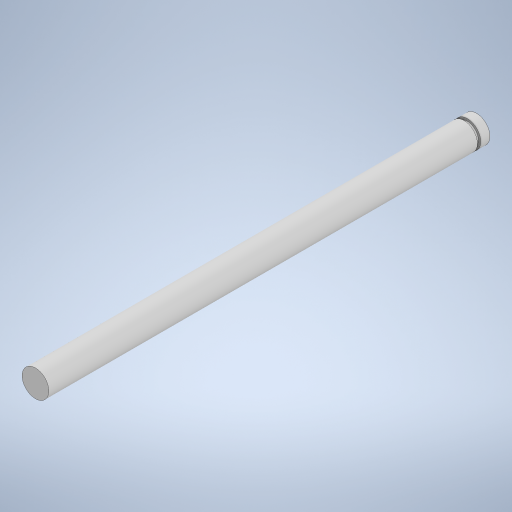
# Autodesk Inventor part: Eixo do Motor Industrial
Saved by Autodesk Inventor 2023 (Build 270158030, 158C)
## iProperties
Created: 2022-07-19
Part Number: Eixo do Motor Industrial
Material: Generic
Document SubType Name: Modeling
Designer: coqui
Density: 1 g/cm^3
Appearance: Default
Author: coqui
Autodesk Inventor part; units mm, degrees
ref_plane "YZ Plane" through (0, 0, 0) normal (1, 0, 0) x (0, 1, 0)
ref_plane "XZ Plane" through (0, 0, 0) normal (0, 1, 0) x (-1, 0, 0)
ref_plane "XY Plane" through (0, 0, 0) normal (0, 0, 1) x (1, 0, 0)
sketch "Sketch1" plane through (0, 0, 0) normal (0, 0, 1) x (1, 0, 0)
  circle A0 centre (0, 0) radius 7.25
  dimension "d0" = 14.5
  constraints: 1 centre point, 1 coincident
  measures "d0" diameter of A0
extrude "Extrusion1" add sketch "Sketch1" along normal blind 240
sketch "Sketch2" plane through (0, 0, 0) normal (0, 1, 0) x (-1, 0, 0)
  line L0 (7.25, 0) -> (7.25, 240) projected
  line L1 (7.25, 5) -> (6, 5)
  line L2 (6, 5) -> (6, 6.8)
  line L3 (6, 6.8) -> (7.25, 6.8)
  line L4 (7.25, 6.8) -> (7.25, 5)
  line L5 (7.25, 0) -> (-7.25, 0) projected
  line L6 (0, 0) -> (0, -34.9846) construction
  dimension "d4" = 1.8
  dimension "d5" = 5
  dimension "d7" = 6
  dimension "d8" = 1.25
  constraints: 10 end point, 2 parallel, 1 horizontal, 1 midpoint, 1 perpendicular, 1 point on line, 1 vertical
  measures "d4" distance of L1.end L2.end
  measures "d5" distance between parallel lines of L5 L1
  measures "d7" distance from line of L6.start L2
  measures "d8" distance of L1.start L1.end
revolve "Revolution1" cut sketch "Sketch2" angle 360 about axis through (0, 0, 0) along (0, 0, -1)
body "Solid1"
